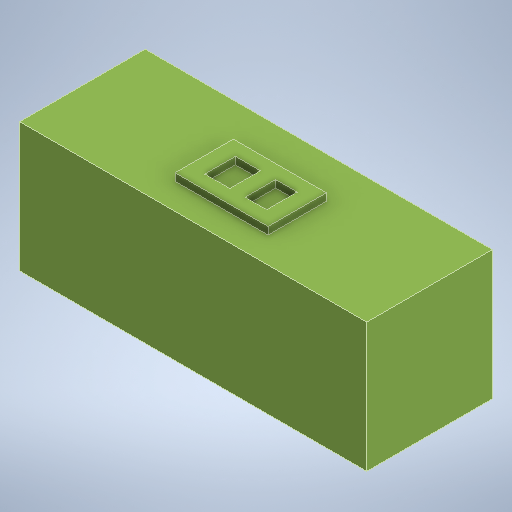
# Autodesk Inventor part: Battery Lipo
Saved by Autodesk Inventor 2025 (Build 290162000, 162)
## iProperties
Created: 2024-08-06
Part Number: Battery Lipo
Material: Generic
Document SubType Name: Modeling
Designer: Pauline Simonnet
Density: 1 g/cm^3
Appearance: Olive Green
Author: Pauline Simonnet
Autodesk Inventor part; units mm, degrees
ref_plane "YZ Plane" through (0, 0, 0) normal (1, 0, 0) x (0, 1, 0)
ref_plane "XZ Plane" through (0, 0, 0) normal (0, 1, 0) x (-1, 0, 0)
ref_plane "XY Plane" through (0, 0, 0) normal (0, 0, 1) x (1, 0, 0)
sketch "Sketch1" plane through (0, 0, 0) normal (0, 1, 0) x (-1, 0, 0)
  line L0 (0, 0) -> (-94, 0)
  line L1 (-94, 0) -> (-94, -34)
  line L2 (-94, -34) -> (0, -34)
  line L3 (0, -34) -> (0, 0)
  dimension "d0" = 34
  dimension "d1" = 94
  constraints: 8 end point, 2 parallel, 1 horizontal, 1 perpendicular
  measures "d0" distance between parallel lines of L2 L0
  measures "d1" distance between parallel lines of L1 L3
extrude "Extrusion1" add sketch "Sketch1" along normal blind 35
sketch "Sketch2" plane through (0, 35, 0) normal (0, 1, 0) x (1, 0, 0)
  line L0 (35.0106, 7.0576) -> (60.2075, 7.0576)
  line L1 (60.2075, 7.0576) -> (60.2075, 10.8183)
  line L2 (60.2075, 10.8183) -> (35.0106, 10.8183)
  line L3 (35.0106, 10.8183) -> (35.0106, 7.0576)
  line L4 (35.0106, 7.0576) -> (39.3355, 7.0576)
  line L5 (39.3355, 7.0576) -> (39.3355, 22.8526)
  line L6 (39.3355, 22.8526) -> (35.0106, 22.8526)
  line L7 (35.0106, 22.8526) -> (35.0106, 7.0576)
  line L8 (35.0106, 22.8526) -> (60.2075, 22.8526)
  line L9 (60.2075, 22.8526) -> (60.2075, 19.0919)
  line L10 (60.2075, 19.0919) -> (35.0106, 19.0919)
  line L11 (35.0106, 19.0919) -> (35.0106, 22.8526)
  line L12 (60.2075, 22.8526) -> (56.0707, 22.8526)
  line L13 (56.0707, 22.8526) -> (56.0707, 7.0576)
  line L14 (56.0707, 7.0576) -> (60.2075, 7.0576)
  line L15 (60.2075, 7.0576) -> (60.2075, 22.8526)
  line L16 (46.1048, 7.0576) -> (50.2416, 7.0576)
  line L17 (50.2416, 7.0576) -> (50.2416, 22.8526)
  line L18 (50.2416, 22.8526) -> (46.1048, 22.8526)
  line L19 (46.1048, 22.8526) -> (46.1048, 7.0576)
  point P0 (0, 0)
  point P1 (39.3355, 10.8183)
  point P2 (39.3355, 19.0919)
  point P3 (46.1048, 19.0919)
  point P4 (46.1048, 10.8183)
  point P5 (50.2416, 19.0919)
  point P6 (56.0707, 19.0919)
  point P7 (56.0707, 10.8183)
  point P8 (50.2416, 10.8183)
  constraints: 40 end point, 10 parallel, 5 horizontal, 5 perpendicular, 4 point on line
extrude "Extrusion2" add sketch "Sketch2" along normal blind 2 contours L3 L2 L5 L0 | L5 L2 L19 L0 | L7 L10 L5 L2 | L19 L2 L17 L0 | L7 L6 L5 L10 | L17 L2 L13 L0 | L19 L10 L17 L2 | L5 L8 L19 L10 | L13 L2 L1 L0 | L19 L8 L17 L10 | L13 L10 L15 L2 | L17 L8 L13 L10 | L13 L8 L9 L10
body "Solid1"
